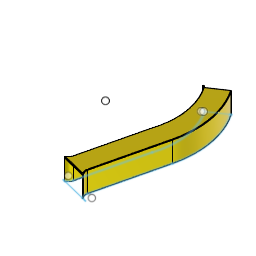
Tunel (Autodesk Fusion 360 design; units mm, degrees)
part number: 2026-05-30-16-29-54-093
Autodesk Fusion 360 part; units mm, degrees
sketch "Sketch1" plane through (0, 0, 0) normal (0, 0, 1) x (1, 0, 0)
  arc A0 (40.8125, 70.866) -> (39.0316, 71.3876) centre (39.6043, 70.0419) ccw
  arc A1 (40.3994, 70.5843) -> (39.3219, 70.962) centre (39.6043, 70.0419) ccw
  arc A2 (45.3863, 40.2197) -> (40.8125, 70.866) centre (11.4188, 50.8147) ccw
  arc A3 (44.9039, 40.3524) -> (40.3994, 70.5843) centre (11.4188, 50.8147) ccw
  line L0 (37.8087, 8.5202) -> (45.3863, 40.2197)
  line L1 (37.3224, 8.6365) -> (44.9039, 40.3524)
  arc A4 (34.9504, 6.3921) -> (37.3224, 8.6365) centre (34.4176, 9.3308) ccw
  arc A5 (35.8752, 6.1635) -> (37.8087, 8.5202) centre (34.4176, 9.3308) ccw
  arc A6 (46.5621, 6.4278) -> (47.4142, 3.3103) centre (49.8315, 5.6462) ccw
  line L2 (54.6994, 40.4687) -> (46.5621, 6.4278)
  arc A7 (55.1857, 40.3524) -> (48.5945, 76.1714) centre (11.4188, 50.8147) ccw
  line L3 (55.1857, 40.3524) -> (47.0484, 6.3115)
  arc A8 (47.0484, 6.3115) -> (49.4188, 2.8147) centre (49.8315, 5.6462) ccw
  arc A9 (54.6994, 40.4687) -> (48.18, 75.8919) centre (11.4188, 50.8147) ccw
  line L4 (39.0316, 71.3876) -> (39.3219, 70.962)
  line L5 (49.4188, 2.8147) -> (47.4142, 3.3103)
  line L6 (34.9504, 6.3921) -> (35.8752, 6.1635)
  line L7 (35.8752, 6.1635) -> (47.4142, 3.3103)
  line L8 (48.18, 75.8919) -> (48.5945, 76.1714)
  line L9 (48.5945, 76.1714) -> (40.7846, 70.9055)
  dimension "d1" = 35
  dimension "d2" = 10
  dimension "d3" = 0.5
  dimension "d4" = 0.5
  constraint tangent L3 A8
  constraint tangent L1 A4
  constraint concentric A6 A8
  constraint concentric A7 A9
  constraint tangent L2 A9
  constraint tangent A6 L2
  constraint concentric A4 A5
  constraint concentric A2 A3
  constraint tangent L0 A5
  constraint tangent A0 A2
  constraint concentric A0 A1
  constraint parallel L5 L6
  constraint parallel L5 L7
  constraint coincident A0 L9.end
  constraint parallel L8 L9
  measures "d1" distance of L3.end A7.start
  measures "d2" distance of L1.start L3.end
  measures "d3" distance of L2 L3
  measures "d4" distance of L0 L1
extrude "Extrude1" add sketch "Sketch1" along normal blind 10.5 contours A0 A1 A2 A3 L0 L1 A4 A5 L4 L6 | A0 A2 L0 A5 A6 L2 A9 L7 L9 | A6 L2 A7 L3 A8 A9 L5 L8 L9
extrude "Extrude2" cut sketch "Sketch1" along normal blind 10 contours A0 A1 A2 A3 L0 L1 A4 A5 L4 L6 | A0 A2 L0 A5 A6 L2 A9 L7 L9 | A6 L2 A7 L3 A8 A9 L5 L8 L9
extrude "Extrude3" add sketch "Sketch1" along normal blind 10 contours A0 A1 A2 A3 L0 L1 A4 A5 L4 L6 | A6 L2 A7 L3 A8 A9 L5 L8 L9
fillet "Fillet1" radius 0.2 8 faces at (49.046, 29.0055, 10.5) (39.8496, 19.2085, 3.5) (36.0166, 6.8083, 7) (46.4714, 52.2383, 7) (40.0271, 70.9065, 7) (52.4733, 29.0055, 7) (54.7333, 63.0152, 7) (48.3714, 3.1853, 7)
